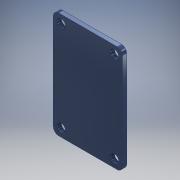
# Autodesk Inventor part: XBee mount
Saved by Autodesk Inventor 2017 (Build 210142000, 142)
## iProperties
Created: 2017-05-18
Part Number: XBee mount
Material: Generic
Document SubType Name: Modeling
Designer: yella
Density: 1 g/cm^3
Appearance: Flaked Satin - Blue
Author: yella
Autodesk Inventor part; units mm, degrees
ref_plane "YZ Plane" through (0, 0, 0) normal (1, 0, 0) x (0, 1, 0)
ref_plane "XZ Plane" through (0, 0, 0) normal (0, 1, 0) x (-1, 0, 0)
ref_plane "XY Plane" through (0, 0, 0) normal (0, 0, 1) x (1, 0, 0)
sketch "Sketch1" plane through (0, 0, 0) normal (0, 1, 0) x (-1, 0, 0)
  line L0 (-13, 18) -> (-13, -18)
  line L1 (-11, -20) -> (11, -20)
  line L2 (13, -18) -> (13, 18)
  line L3 (11, 20) -> (-11, 20)
  arc A0 (13, 18) -> (11, 20) centre (11, 18) ccw
  arc A1 (11, -20) -> (13, -18) centre (11, -18) ccw
  arc A2 (-13, -18) -> (-11, -20) centre (-11, -18) ccw
  arc A3 (-11, 20) -> (-13, 18) centre (-11, 18) ccw
  line L4 (11, 20) -> (13, 20)
  line L5 (13, 20) -> (13, 17)
  line L6 (13, 17) -> (10, 17)
  circle A4 centre (10, 17) radius 1.6
  line L7 (-13, 20) -> (-13, 17)
  line L8 (-13, 17) -> (-10, 17)
  circle A5 centre (-10, 17) radius 1.6
  line L9 (13, -20) -> (10, -20)
  line L10 (10, -20) -> (10, -17)
  line L11 (-13, -20) -> (-10, -20)
  line L12 (-10, -20) -> (-10, -17)
  circle A6 centre (10, -17) radius 1.6
  circle A7 centre (-10, -17) radius 1.6
  dimension "d2" = 2
  dimension "d6" = 3
  dimension "d7" = 3
  dimension "d8" = 3.2
  dimension "d9" = 3
  dimension "d10" = 3
  dimension "d11" = 3.2
  dimension "d12" = 3
  dimension "d13" = 3
  dimension "d14" = 3
  dimension "d15" = 3
  dimension "d16" = 3.2
  dimension "d17" = 3.2
  constraints: 26 end point, 8 centre point, 8 point on circle, 8 tangent, 5 perpendicular, 5 point on line, 4 coincident, 3 equal radius, 2 parallel, 1 horizontal, 1 vertical
  measures "d2" radius of A0
  measures "d6" distance of L4.end L5.end
  measures "d7" distance of L5.end L6.end
  measures "d8" diameter of A4
  measures "d9" distance of L7.start L7.end
  measures "d10" distance of L7.end L8.end
  measures "d11" diameter of A5
  measures "d12" distance of L9.start L9.end
  measures "d13" distance of L9.end L10.end
  measures "d14" distance of L11.start L11.end
  measures "d15" distance of L11.end L12.end
  measures "d16" diameter of A6
  measures "d17" diameter of A7
extrude "Extrusion1" add sketch "Sketch1" along normal blind 1.6 contours A3 L3 A0 L2 A1 L1 A2 L0
body "Solid1"
